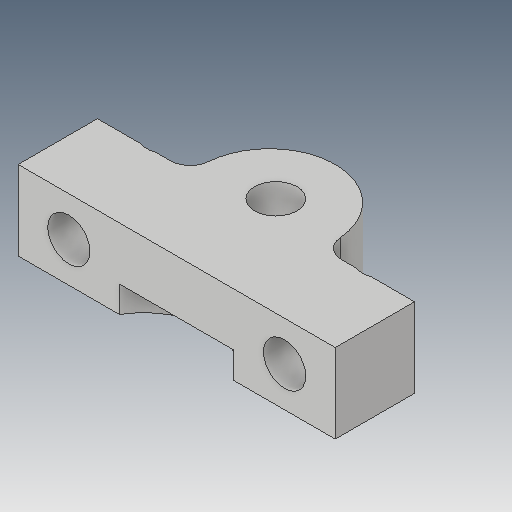
# Autodesk Inventor part: DfixPit
Saved by Autodesk Inventor 2019.4 (Build 234330000, 330)
## iProperties
Created: 2019-06-16
Part Number: DfixPit
Material: Generic
Document SubType Name: Modeling
Designer: AzLIer
Density: 1 g/cm^3
Appearance: Default
Mass: 0.989234 g
Surface Area: 9.23002 cm^2
Volume: 0.989234 cm^3
Author: AzLIer
Autodesk Inventor part; units mm, degrees
ref_plane "YZ Plane" through (0, 0, 0) normal (1, 0, 0) x (0, 1, 0)
ref_plane "XZ Plane" through (0, 0, 0) normal (0, 1, 0) x (-1, 0, 0)
ref_plane "XY Plane" through (0, 0, 0) normal (0, 0, 1) x (1, 0, 0)
sketch "スケッチ1" plane through (0, 0, 0) normal (0, 0, 1) x (1, 0, 0)
  line L0 (12, -3) -> (-12, -3)
  line L1 (-12, -3) -> (-12, 3)
  line L2 (-12, 3) -> (12, 3)
  line L3 (12, 3) -> (12, -3)
  line L4 (12, -3) -> (-12, 3) construction
  line L5 (-12, -3) -> (12, 3) construction
  point P0 (0, 0)
  dimension "d0" = 24
  dimension "d1" = 6
  constraints: 12 end point, 2 midpoint, 2 parallel, 1 horizontal, 1 perpendicular
  measures "d0" distance of L1.end L2.end
  measures "d1" distance of L0.end L1.end
extrude "押し出し1" add sketch "スケッチ1" along normal blind 20
sketch "スケッチ2" plane through (-12, -3, 0) normal (0, -1, 0) x (1, 0, 0)
  line L0 (23.1845, 35.5) -> (0.8155, 35.5) projected
  arc A0 (0.8155, 35.5) -> (-4.2691, 17.077) centre (12, 22.5) ccw projected
  arc A1 (-4.2691, 17.077) -> (0, 14) centre (0, 18.5) ccw projected
  line L1 (0, 14) -> (0, 17) projected
  arc A2 (0, 20) -> (0, 17) centre (0, 18.5) ccw projected
  line L2 (0, 20) -> (3.2964, 20) projected
  arc A3 (4.3735, 20) -> (3.2964, 20) centre (3.8349, 18.6) ccw projected
  line L3 (4.3735, 20) -> (7.6699, 20) projected
  arc A4 (16.3301, 20) -> (7.6699, 20) centre (12, 22.5) ccw projected
  line L4 (16.3301, 20) -> (19.6265, 20) projected
  arc A5 (20.7036, 20) -> (19.6265, 20) centre (20.1651, 18.6) ccw projected
  line L5 (20.7036, 20) -> (24, 20) projected
  arc A6 (24, 17) -> (24, 20) centre (24, 18.5) ccw projected
  line L6 (24, 17) -> (24, 14) projected
  arc A7 (24, 14) -> (28.2691, 17.077) centre (24, 18.5) ccw projected
  arc A8 (28.2691, 17.077) -> (23.1845, 35.5) centre (12, 22.5) ccw projected
  circle A9 centre (25, 24.5) radius 1.6 projected
  circle A10 centre (12, 32.5) radius 1.6 projected
  circle A11 centre (-1, 24.5) radius 1.6 projected
  line L7 (24, 0) -> (0, 0) projected
  line L8 (24, 0) -> (24, 14)
  line L9 (0, 20) -> (24, 20) projected
  circle A12 centre (12, 12.5) radius 1.6
  arc A13 (7.0148, 12.6154) -> (16.9852, 12.6154) centre (12, 13) ccw
  line L10 (3.8349, 18.6) -> (3.8349, 14) construction
  line L11 (20.1651, 18.6) -> (20.1651, 14) construction
  line L12 (0, 14) -> (5.5193, 14)
  line L13 (18.4807, 14) -> (24, 14)
  arc A14 (4.3735, 14) -> (3.2964, 14) centre (3.8349, 12.6) ccw
  arc A15 (20.7036, 14) -> (19.6265, 14) centre (20.1651, 12.6) ccw
  line L14 (5.3349, 18.6) -> (5.3349, 14) construction
  line L15 (18.6651, 18.6) -> (18.6651, 14) construction
  arc A16 (7.0148, 12.6154) -> (5.5193, 14) centre (5.5193, 12.5) ccw
  arc A17 (18.4807, 14) -> (16.9852, 12.6154) centre (18.4807, 12.5) ccw
  line L16 (0, 0) -> (0, 14)
  point P0 (12, 0)
  point P1 (7.101, 14)
  point P2 (16.899, 14)
  point P3 (12, 8)
  dimension "d5" = 3.2
  dimension "d6" = 10
  dimension "d7" = 4.5
  dimension "d8" = 5
  dimension "d11" = 3
  dimension "d12" = 3
  dimension "d13" = 1.4
  dimension "d14" = 1.5
  dimension "d15" = 1.5
  dimension "d16" = 1.5
  constraints: 16 end point, 15 point on circle, 10 point on line, 6 centre point, 4 perpendicular, 4 tangent, 2 horizontal, 2 parallel, 2 vertical alignment, 1 collinear, 1 equal radius, 1 horizontal alignment
  measures "d5" diameter of A12
  measures "d6" distance of A0.centre A12.centre
  measures "d7" distance of A12.centre point (12, 8)
  measures "d8" radius of A13
  measures "d11" diameter of A14
  measures "d12" diameter of A15
  measures "d13" distance from line of L12 A14.centre
  measures "d14" distance between parallel lines of L10 L14
  measures "d15" distance between parallel lines of L11 L15
  measures "d16" radius of A16
extrude "押し出し2" cut sketch "スケッチ2" against normal through all contours L8 L7 L16 L12 A16 A13 A17 L13 | L13 A15 | A14 L12 | A12
sketch "スケッチ3" plane through (-12, -3, 20) normal (0, -1, 0) x (1, 0, 0)
  arc A0 (16.3301, 0) -> (7.6699, 0) centre (12, 2.5) ccw projected
  circle A1 centre (12, 2.5) radius 5
  point P0 (12, -20)
  dimension "d19" = 10
  constraints: 1 centre point, 1 coincident
  measures "d19" diameter of A1
extrude "押し出し3" cut sketch "スケッチ3" against normal blind 2
sketch "スケッチ4" plane through (0, 0, 20) normal (0, 0, 1) x (1, 0, 0)
  circle A0 centre (8.1651, 0) radius 1.2295 projected
  circle A1 centre (-8.1651, 0) radius 1.2295 projected
  line L0 (-11.1845, 3) -> (11.1845, 3) projected
  line L1 (-11.1845, -3) -> (-11.1845, 3) projected
  line L2 (11.1845, -3) -> (-11.1845, -3) projected
  line L3 (11.1845, 3) -> (11.1845, -3) projected
  point P0 (0, 0)
hole "穴1" at (-8.1651, 0, 20) at (8.1651, 0, 20) direction (0, 0, -1) diameter 3.2 end through all
